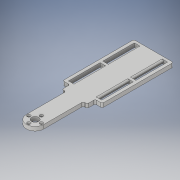
# Autodesk Inventor part: arm2
Saved by Autodesk Inventor 2019 (Build 230136000, 136)
## iProperties
Created: 2018-10-22
Part Number: arm2
Material: 일반
Document SubType Name: Modeling
Designer: otm09
Density: 1 g/cm^3
Appearance: 기본값
Mass: 34.0103 g
Surface Area: 181.28 cm^2
Volume: 34.0103 cm^3
Author: otm09
Autodesk Inventor part; units mm, degrees
ref_plane "YZ Plane" through (0, 0, 0) normal (1, 0, 0) x (0, 1, 0)
ref_plane "XZ Plane" through (0, 0, 0) normal (0, 1, 0) x (-1, 0, 0)
ref_plane "XY Plane" through (0, 0, 0) normal (0, 0, 1) x (1, 0, 0)
sketch "스케치1" plane through (0, 0, 0) normal (0, 1, 0) x (-1, 0, 0)
  circle A0 centre (0, 0) radius 11
  circle A1 centre (0, -8) radius 1.1
  circle A2 centre (0, 0) radius 11
  circle A3 centre (8, 0) radius 1.1
  circle A4 centre (0, 0) radius 11
  circle A5 centre (0, 8) radius 1.1
  circle A6 centre (0, 0) radius 11
  circle A7 centre (-8, 0) radius 1.1
  line L0 (-11, 0) -> (-11, -150)
  line L1 (-11, -150) -> (11, -150)
  line L2 (11, -150) -> (11, 0)
  line L3 (16, -150) -> (-16, -150)
  line L4 (-16, -150) -> (-16, -50)
  line L5 (-16, -50) -> (16, -50)
  line L6 (16, -50) -> (16, -150)
  arc A8 (-11, 0) -> (11, 0) centre (0, 0) ccw
  circle A9 centre (0, 0) radius 4.5
  line L7 (25, -150) -> (-25, -150)
  line L8 (-25, -150) -> (-25, -60)
  line L9 (-25, -60) -> (25, -60)
  line L10 (25, -60) -> (25, -150)
  line L11 (16, -63.3333) -> (21, -63.3333)
  line L12 (21, -63.3333) -> (21, -103.3333)
  line L13 (21, -103.3333) -> (16, -103.3333)
  line L14 (16, -103.3333) -> (16, -63.3333)
  line L15 (16, -106.6667) -> (21, -106.6667)
  line L16 (21, -106.6667) -> (21, -146.6667)
  line L17 (21, -146.6667) -> (16, -146.6667)
  line L18 (16, -146.6667) -> (16, -106.6667)
  line L19 (-16, -63.3333) -> (-21, -63.3333)
  line L20 (-21, -63.3333) -> (-21, -103.3333)
  line L21 (-21, -103.3333) -> (-16, -103.3333)
  line L22 (-16, -103.3333) -> (-16, -63.3333)
  line L23 (-16, -106.6667) -> (-21, -106.6667)
  line L24 (-21, -106.6667) -> (-21, -146.6667)
  line L25 (-21, -146.6667) -> (-16, -146.6667)
  line L26 (-16, -146.6667) -> (-16, -106.6667)
  dimension "d1" = 2.2
  dimension "d5" = 360
  dimension "d7" = 150
  dimension "d8" = 32
  dimension "d9" = 100
  dimension "d24" = 9
  dimension "d26" = 50
  dimension "d27" = 90
  dimension "d28" = 9
  dimension "d29" = 5
  dimension "d30" = 40
  dimension "d31" = 5
  dimension "d32" = 40
  dimension "d33" = 3.3333
  dimension "d34" = 3.3333
  dimension "d35" = 5
  dimension "d36" = 40
  dimension "d37" = 5
  dimension "d38" = 40
  dimension "d39" = 3.3333
  dimension "d40" = 3.3333
  constraints: 54 end point, 13 parallel, 9 centre point, 6 horizontal, 6 perpendicular, 4 point on line, 3 coincident, 2 coincident with centre, 2 collinear, 2 point on circle, 1 horizontal alignment, 17 other
  measures "d1" diameter of A1
  measures "d7" distance of L0.end L0.start
  measures "d8" distance of L4.end L5.end
  measures "d9" distance of L3.end L4.end
  measures "d24" diameter of A9
  measures "d26" distance of L8.end L9.end
  measures "d27" distance of L7.end L8.end
  measures "d28" distance between parallel lines of L6 L10
  measures "d29" distance of L12.end L13.end
  measures "d30" distance of L11.end L12.end
  measures "d31" distance of L16.end L17.end
  measures "d32" distance of L15.end L16.end
  measures "d33" distance between parallel lines of L9 L11
  measures "d34" distance between parallel lines of L15 L13
  measures "d35" distance of L21.end L20.end
  measures "d36" distance of L20.end L19.end
  measures "d37" distance of L25.end L24.end
  measures "d38" distance of L24.end L23.end
  measures "d39" distance between parallel lines of L9 L19
  measures "d40" distance between parallel lines of L23 L21
extrude "돌출1" add sketch "스케치1" along normal blind 5 contours A0 | L2 L5 L0 A0 | L5 L6 L9 L2 | L2 L9 L0 L5 | L0 L9 L4 L5 | L9 L6 L3 L2 | L2 L1 L0 L9 | L0 L3 L4 L9 | L9 L10 L7 L6 L17 L16 L15 L13 L12 L11 | L4 L19 L20 L21 L23 L24 L25 L7 L8 L9
fillet "모깎기1" radius 2 18 edges at (16, 5, -83.3333) (16, 5, -126.6667) (16, 0, -126.6667) (16, 0, -83.3333) (-16, 5, -83.3333) (-16, 5, -126.6667) (16, 2.5, -50) (25, 2.5, -60) (16, 2.5, -60) (11, 2.5, -50) (-11, 2.5, -50) (-16, 2.5, -50) (-16, 2.5, -60) (-25, 2.5, -60) (-16, 0, -83.3333) (-16, 0, -126.6667) (25, 2.5, -150) (-25, 2.5, -150)
sketch "스케치2" plane through (0, 5, 0) normal (0, 1, 0) x (1, 0, 0)
  circle A0 centre (-8, 0) radius 1.1 projected
  circle A1 centre (-8, 0) radius 2.1
  circle A2 centre (0, -8) radius 2.1
  circle A3 centre (8, 0) radius 2.1
  circle A4 centre (0, 8) radius 2.1
  point P0 (0, 0)
  dimension "d42" = 4.2
  dimension "d45" = 360
  constraints: 4 centre point, 1 coincident, 9 other
  measures "d42" diameter of A1
extrude "돌출2" cut sketch "스케치2" against normal blind 2
equation "\"d28\" = -0.5 * d8 + 0.5 * d26"
equation "\"d31\" = d29"
equation "\"d32\" = d30"
equation "\"d33\" = -0.333333 * d30 + 0.333333 * d27 - 0.333333 * d32"
equation "\"d34\" = -0.333333 * d30 + 0.333333 * d27 - 0.333333 * d32"
equation "\"d35\" = d29"
equation "\"d36\" = d30"
equation "\"d37\" = d29"
equation "\"d38\" = d30"
equation "\"d39\" = -0.333333 * d30 + 0.333333 * d27 - 0.333333 * d32"
equation "\"d40\" = -0.333333 * d30 + 0.333333 * d27 - 0.333333 * d32"
